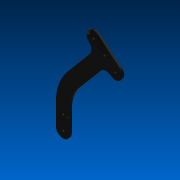
# Autodesk Inventor part: Hood Upper Bracket
Saved by Autodesk Inventor 2022 (Build 260153000, 153)
## iProperties
Created: 2022-04-17
Part Number: Hood Upper Bracket
Material: PET Plastic
Document SubType Name: Modeling
Designer: omard
Density: 1.541 g/cm^3
Appearance: Smooth - Black
Author: omard
Autodesk Inventor part; units mm, degrees
ref_plane "YZ Plane" through (0, 0, 0) normal (1, 0, 0) x (0, 1, 0)
ref_plane "XZ Plane" through (0, 0, 0) normal (0, 1, 0) x (-1, 0, 0)
ref_plane "XY Plane" through (0, 0, 0) normal (0, 0, 1) x (1, 0, 0)
sketch "Sketch1" plane through (0, 0, 0) normal (0, 0, 1) x (1, 0, 0)
  line L0 (-12.7, 25.4) -> (12.7, 25.4)
  line L1 (12.7, 25.4) -> (12.7, -25.4)
  line L2 (12.7, -25.4) -> (-12.7, -25.4)
  line L3 (-12.7, -25.4) -> (-12.7, 25.4)
  line L4 (-12.7, 25.4) -> (12.7, -25.4) construction
  line L5 (12.7, 25.4) -> (-12.7, -25.4) construction
  line L6 (72.5658, 158.7842) -> (111.4809, 126.1305)
  line L7 (111.4809, 126.1305) -> (95.1541, 106.673)
  line L8 (95.1541, 106.673) -> (56.239, 139.3266)
  line L9 (56.239, 139.3266) -> (72.5658, 158.7842)
  line L10 (72.5658, 158.7842) -> (95.1541, 106.673) construction
  line L11 (111.4809, 126.1305) -> (56.239, 139.3266) construction
  line L12 (74.1312, 140.892) -> (93.5887, 124.5652) construction
  line L13 (0, -12.7) -> (0, 12.7) construction
  line L14 (-12.7, -25.4) -> (12.7, -25.4)
  line L15 (12.7, -25.4) -> (12.7, -50.8)
  line L16 (12.7, -50.8) -> (-12.7, -50.8)
  line L17 (-12.7, -50.8) -> (-12.7, -25.4)
  circle A0 centre (0, -38.1) radius 12.7
  line L18 (75.6966, 122.9998) -> (56.239, 139.3266)
  line L19 (56.239, 139.3266) -> (-17.8482, 51.033)
  line L20 (-17.8482, 51.033) -> (1.6094, 34.7061)
  line L21 (1.6094, 34.7061) -> (75.6966, 122.9998)
  line L22 (72.5658, 158.7842) -> (56.239, 139.3266)
  line L23 (56.239, 139.3266) -> (36.7815, 155.6534)
  line L24 (36.7815, 155.6534) -> (53.1083, 175.111)
  line L25 (53.1083, 175.111) -> (72.5658, 158.7842)
  line L26 (54.6737, 157.2188) -> (74.1312, 140.892) construction
  arc A1 (62.8371, 166.9476) -> (46.5103, 147.49) centre (54.6737, 157.2188) ccw
  circle A2 centre (93.5887, 124.5652) radius 12.7
  line L27 (192.4417, 25.039) -> (17.324, 171.9802)
  circle A3 centre (0, -12.7) radius 12.7
  arc A4 (7.7203, 81.5042) -> (-12.7, 25.4) centre (74.5827, 25.4) ccw
  arc A5 (27.1778, 65.1774) -> (12.7, 25.4) centre (74.5827, 25.4) ccw
  point P0 (0, 0)
  point P1 (0, 0)
  point P2 (0, 0)
  point P3 (83.86, 132.7286)
  point P4 (83.86, 132.7286)
  point P5 (-12.7, -38.1)
  point P6 (12.7, -38.1)
  point P7 (-12.7, -4.4935)
  point P8 (12.7, -4.4935)
  point P9 (75.6966, 122.9998)
  point P10 (85.4253, 114.8364)
  point P11 (101.7521, 134.294)
  point P12 (-12.7, -12.7)
  point P13 (12.7, -12.7)
  dimension "d0" = 25.4
  dimension "d1" = 50.8
  dimension "d2" = 25.4
  dimension "d3" = 12.7
  dimension "d17" = 127
  constraints: 56 end point, 11 parallel, 10 midpoint, 9 tangent, 7 collinear, 7 equal length, 6 centre point, 6 point on circle, 5 perpendicular, 5 point on line, 4 coincident, 2 horizontal, 2 vertical alignment, 1 vertical, 3 other
  measures "d0" distance between parallel lines of L3 L1
  measures "d1" distance between parallel lines of L2 L0
  measures "d2" distance of L13.start L13.end
  measures "d3" distance of L13.start point (0, 0)
  measures "d17" distance from line of L27.start L7
extrude "Extrusion1" add sketch "Sketch1" along normal blind 3.175 contours A4 L20 L21 A5 L0 | L0 L1 A3 L3 | A3 | A4 L19 L8 L21 L20 | L8 L9 L6 A2 | L23 A1 L25 L9 | A2
hole "Hole1" at (0, -12.7, 0) at (0, 12.7, 0) at (93.5887, 124.5652, 0) at (74.1312, 140.892, 0) at (0, -38.1, 0) at (54.6737, 157.2188, 0) direction (0, 0, 1) diameter 4.445 end through all
fillet "Fillet1" radius 12.7 2 edges at (56.239, 139.3266, 1.5875) (75.6966, 122.9998, 1.5875)
equation "\"d3\" = 0.5 * d2"
body "Solid1"
